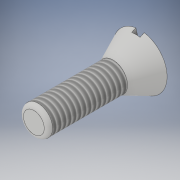
# Autodesk Inventor part: Screw
Saved by Autodesk Inventor 2019 (Build 230136000, 136)
## iProperties
Created: 2019-02-03
Part Number: Screw
Material: Generic
Document SubType Name: Modeling
Designer: Jared
Density: 1 g/cm^3
Appearance: Default
Author: Jared
Autodesk Inventor part; units mm, degrees
ref_plane "YZ Plane" through (0, 0, 0) normal (1, 0, 0) x (0, 1, 0)
ref_plane "XZ Plane" through (0, 0, 0) normal (0, 1, 0) x (-1, 0, 0)
ref_plane "XY Plane" through (0, 0, 0) normal (0, 0, 1) x (1, 0, 0)
sketch "Sketch1" plane through (0, 0, 0) normal (0, 1, 0) x (-1, 0, 0)
  line L0 (0, 0) -> (0, 13.5)
  line L1 (0, 13.5) -> (1.75, 13.5)
  line L2 (1.75, 13.5) -> (1.75, 4)
  line L3 (0, 0) -> (3.25, 0.75)
  line L4 (1.75, 4) -> (3.25, 0.75)
  dimension "d0" = 13.5
  dimension "d1" = 1.75
  dimension "d2" = 3.25
  dimension "d4" = 0.75
  dimension "d5" = 9.5
  constraints: 10 end point, 2 perpendicular, 1 coincident, 1 vertical
  measures "d0" distance of L0.start L0.end
  measures "d1" distance of L0.end L1.end
  measures "d2" distance from line of L0 L3.end
  measures "d4" vertical distance of L0.start L3.end
  measures "d5" distance of L1.end L2.end
revolve "Revolution1" add sketch "Sketch1" angle 360 about axis through (0, 0, 0) along (0, 0, 1)
ref_plane "Work Plane1" through (0, 0, 0) normal (0, 0, 1) x (1, 0, 0)
sketch "Sketch2" plane through (0, 0, 0) normal (0, 0, 1) x (1, 0, 0)
  line L0 (0.5, 3.2113) -> (0.5, -3.2113)
  line L1 (-0.5, 3.2113) -> (-0.5, -3.2113)
  circle A0 centre (0, 0) radius 3.25 projected
  dimension "d8" = 1
  dimension "d9" = 0.5
  constraints: 4 end point, 4 point on circle, 2 vertical
  measures "d8" distance between parallel lines of L0 L1
  measures "d9" distance from line of L1 point (0, 0)
extrude "Extrusion1" cut sketch "Sketch2" along normal blind 1.25 contours L0 A0 L1
thread "Thread1" size "M3.5x0.6" class "6g" standard "ANSI Metric M Profile" full length
fillet "Fillet1" radius 0.5 1 edges at (1.75, 0, 13.5)
body "Solid1"
